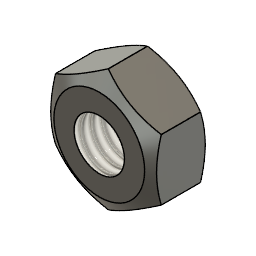
_D6H5TS5AVR8F43N3R1XL613M4en-US11.c9319d48-3e45-4f47-b580-171f8668bec4 (Autodesk Fusion 360 design; units mm, degrees)
description: Hex Nut Style 2 ANSI B18.2.4.2M - M4x0.7
part number: HNS2 ANSI B18.2.4.2M - M4x0.7 Steel Grade 2H Plain
Autodesk Fusion 360 part; units mm, degrees
sketch "Sketch1" plane through (0, 0, 0) normal (0, 1, 0) x (1, 0, 0)
  line L0 (0, 0) -> (0, -3.8)
  line L1 (-2, 0) -> (-3, 0)
  line L2 (-3, 0) -> (-4.04, -0.6004)
  line L3 (-4.04, -0.6004) -> (-4.04, -3.1996)
  line L4 (-4.04, -3.1996) -> (-3, -3.8)
  line L5 (-3, -3.8) -> (-2, -3.8)
  line L6 (-2, -3.8) -> (-2, 0)
  dimension "d121" = 4
  dimension "d122" = 30
  dimension "d123" = 30
  dimension "d125" = 6
  dimension "d128" = 8.08
  dimension "d153" = 3.8
  constraint vertical L0
  constraint coincident L0 L0.end
  constraint coincident origin L0
  constraint coincident L0.start L1
  constraint coincident L0.start origin
  constraint vertical L1.end L4.end
  constraint coincident L0.end L5
  constraint horizontal L1
  measures "d122" angle of L1 L2
  measures "d123" angle of L4 L5
  measures "d153" distance of L1 L5
revolve "Revolve1" add sketch "Sketch1" angle 360 about axis through (0, 0, 0) along (0, 0, 1)
sketch "Sketch8" plane through (0, 0, 3.8) normal (0, 0, 1) x (1, 0, 0)
  line L0 (-3.5, -2.0178) -> (-3.5, 2.0178)
  circle A0 centre (0, 0) radius 2
  circle A1 centre (0, 0) radius 4.04
  dimension "d114" = 3.5
  constraint coincident L0.end A1
  constraint coincident L0.start A1
  constraint vertical L0
  measures "d114" distance of A0.centre L0
extrude "Extrude5" cut sketch "Sketch8" against normal blind 3.8 contours L0 A1 picked at (-3.5871, 0.4914)
pattern_circular "C-Pattern2" count 6 over 360 about axis through (0, 0, 1.75) along (0, 0, 1) of "Extrude5"
thread "Thread3" "ANSI Metric M Profile 4.0 M4x0.7 M4x0.7 6H" major diameter 4.1095 minor diameter 3.332 pitch 0.7 angle 60 resizes the face on face at (-1.9901, 0.1991, 2.5333)
equation "adsk_nheig = 3.80 mm"
equation "adsk_maxdia = 8.08 mm"
equation "adsk_nomdia = 4.00 mm"
equation "d89 = -adsk_nheig"
equation "adsk_waflat = 7.00 mm"
equation "d114 = adsk_waflat / 2"
equation "adsk_chamang1 = 30 deg"
equation "adsk_chamang2 = 30 deg"
equation "d121 = adsk_nomdia"
equation "d122 = adsk_chamang1"
equation "d123 = adsk_chamang2"
equation "d125 = adsk_beardia"
equation "d128 = adsk_maxdia"
equation "d147 = adsk_nheig"
equation "adsk_beardia = 6.00 mm"
equation "d153 = adsk_nheig"
